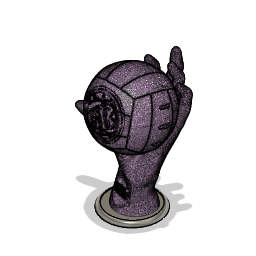
Trofeo Pelota GB (Autodesk Fusion 360 design; units mm, degrees)
Autodesk Fusion 360 part; units mm, degrees
sketch "Sketch2" plane through (0, 0, 0) normal (0, 1, 0) x (1, 0, 0)
  circle A0 centre (0, 0) radius 25
  circle A1 centre (0, 0) radius 21.5
  dimension "d1" = 50
  dimension "d2" = 43
  constraint coincident A0.centre A1.centre
  constraint concentric A0 A1
  measures "d1" diameter of A0
  measures "d2" diameter of A1
extrude "Extrude1" add sketch "Sketch2" along normal blind 3.7
extrude "Extrude2" add sketch "Sketch2" along normal blind 3 contours A1
sketch "Sketch3" plane through (0, 0, 0) normal (1, 0, 0) x (0, 0, -1)
  line L0 (25, 0) -> (-25, 0)
  line L1 (25, 3.7) -> (-25, 3.7)
  circle A0 centre (-21.3, 0) radius 3.7
  line L2 (-25, 0) -> (-25, 3.7)
  constraint tangent L1 A0
  constraint coincident L0 A0.centre
  constraint coincident L0.end L2.start
  constraint coincident L1.end L2.end
  constraint tangent A0 L2
revolve "Revolve1" cut sketch "Sketch3" angle 360 about axis through (0, 1.75, 0) along (0, 1, 0) contours L1 A0 L2
mesh "Mesh1" [no effect]
sketch "Sketch4" plane through (0, 0, 0) normal (0, 1, 0) x (1, 0, 0)
